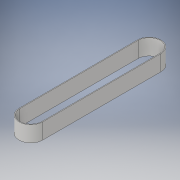
# Autodesk Inventor part: 0nhk
Saved by Autodesk Inventor 2019 (Build 230136000, 136)
## iProperties
Created: 2021-12-23
Part Number: 0nhk
Material: 一般
Document SubType Name: Sheet Metal
Designer: yuta
Density: 1 g/cm^3
Sheet Metal Rule: Default_mm
Appearance: 既定
Author: yuta
Autodesk Inventor part; units mm, degrees
ref_plane "YZ Plane" through (0, 0, 0) normal (1, 0, 0) x (0, 1, 0)
ref_plane "XZ Plane" through (0, 0, 0) normal (0, 1, 0) x (-1, 0, 0)
ref_plane "XY Plane" through (0, 0, 0) normal (0, 0, 1) x (1, 0, 0)
sketch "スケッチ1" plane through (0, 0, 0) normal (0, 1, 0) x (-1, 0, 0)
  line L0 (0, 109.6209) -> (0, -190.3791) construction
  line L1 (-30, 109.6209) -> (-30, -190.3791)
  line L2 (30, -190.3791) -> (30, 109.6209)
  arc A0 (30, 109.6209) -> (-30, 109.6209) centre (0, 109.6209) ccw
  arc A1 (-30, -190.3791) -> (30, -190.3791) centre (0, -190.3791) ccw
  line L3 (0, 109.6209) -> (0, -190.3791) construction
  line L4 (-28.13, 109.6209) -> (-28.13, -190.3791)
  line L5 (28.13, -190.3791) -> (28.13, 109.6209)
  arc A2 (28.13, 109.6209) -> (-28.13, 109.6209) centre (0, 109.6209) ccw
  arc A3 (-28.13, -190.3791) -> (28.13, -190.3791) centre (0, -190.3791) ccw
  point P0 (0, 0)
  point P1 (0, -40.3791)
  point P2 (0, -40.3791)
  dimension "d0" = 300
  dimension "d1" = 60
  dimension "d2" = 56.26
  constraints: 16 end point, 8 point on circle, 8 tangent, 4 centre point, 3 equal length, 2 midpoint, 1 vertical
  measures "d0" distance of L0.start L0.end
  measures "d1" diameter of A1
  measures "d2" diameter of A3
extrude "押し出し1" add sketch "スケッチ1" along normal blind 40
equation "\"BendRadius\" = Thickness"
equation "\"BendReliefWidth\" = Thickness"
equation "\"BendReliefDepth\" = 0.5 * Thickness"
equation "\"CornerReliefSize\" = 4 * Thickness"
equation "\"MinimumRemnant\" = 2 * Thickness"
equation "\"TransitionRadius\" = BendRadius"
equation "\"JacobiRadiusSize\" = BendRadius"
equation "\"GapSize\" = Thickness"
equation "\"Thickness\" = 0.5"
